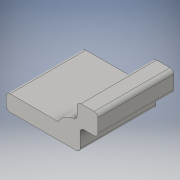
# Autodesk Inventor part: Igus Slider
Saved by Autodesk Inventor 2016 (Build 200138000, 138)
## iProperties
Created: 2016-02-14
Part Number: Igus Slider
Material: Generic
Document SubType Name: Modeling
Designer: Margret
Density: 1 g/cm^3
Appearance: Default
Author: Margret
Autodesk Inventor part; units mm, degrees
ref_plane "YZ Plane" through (0, 0, 0) normal (1, 0, 0) x (0, 1, 0)
ref_plane "XZ Plane" through (0, 0, 0) normal (0, 1, 0) x (-1, 0, 0)
ref_plane "XY Plane" through (0, 0, 0) normal (0, 0, 1) x (1, 0, 0)
sketch "Sketch1" plane through (0, 0, 0) normal (0, 0, 1) x (1, 0, 0)
  line L0 (0, 0) -> (24.765, 0)
  line L1 (24.765, 0) -> (24.765, 5.3594)
  line L2 (24.765, 5.3594) -> (0, 5.3594)
  line L3 (0, 5.3594) -> (0, 0)
  line L4 (23.7236, 7.3152) -> (30.734, 7.3152)
  line L5 (30.734, 7.3152) -> (30.734, 14.3256)
  line L6 (30.734, 14.3256) -> (23.7236, 14.3256)
  line L7 (23.7236, 14.3256) -> (23.7236, 7.3152)
  arc A0 (23.7236, 8.9916) -> (17.4244, 5.3594) centre (23.7236, 1.7133) ccw
  line L8 (24.765, 5.3594) -> (24.765, 7.3152)
  dimension "d0" = 24.765
  dimension "d1" = 5.3594
  dimension "d2" = 30.734
  dimension "d3" = 7.0104
  dimension "d4" = 14.3256
  dimension "d5" = 17.4244
  dimension "d6" = 5.334
  constraints: 18 end point, 4 parallel, 3 perpendicular, 3 point on line, 2 horizontal, 2 point on circle, 1 centre point, 1 vertical, 1 vertical alignment
  measures "d0" distance of L0.start L0.end
  measures "d1" distance of L2.end L0.start
  measures "d2" distance between parallel lines of L5 L3
  measures "d3" distance of L5.end L6.end
  measures "d4" distance between parallel lines of L6 L0
  measures "d5" distance of L2.end A0.end
  measures "d6" distance from line of A0.start L6
extrude "Extrusion1" add sketch "Sketch1" along normal blind 25.4
fillet "Fillet1" radius 1.27 1 edges at (30.734, 14.3256, 12.7)
fillet "Fillet2" radius 1.27 2 edges at (30.734, 7.3152, 12.7) (23.7236, 14.3256, 12.7)
fillet "Fillet3" radius 1.27 5 edges at (23.7236, 8.9916, 12.7) (24.765, 7.3152, 12.7) (24.765, 0, 12.7) (0, 0, 12.7) (0, 5.3594, 12.7)
body "Solid1"
